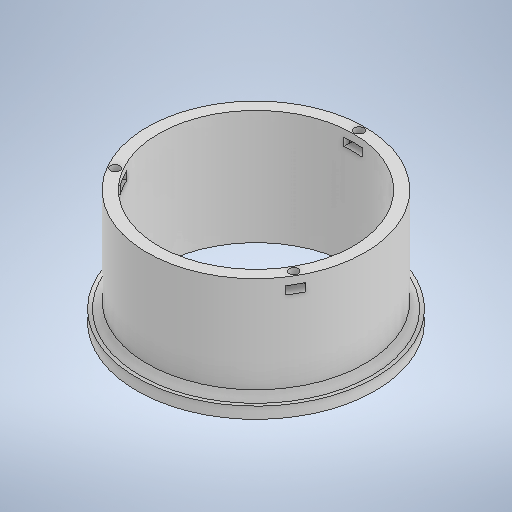
# Autodesk Inventor part: Center Cylinder
Saved by Autodesk Inventor 2025 (Build 290162000, 162)
## iProperties
Created: 2025-07-09
Part Number: Center Cylinder
Material: Generic
Document SubType Name: Modeling
Designer: mumin
Density: 1 g/cm^3
Appearance: Default
Author: mumin
Autodesk Inventor part; units mm, degrees
ref_plane "YZ Plane" through (0, 0, 0) normal (1, 0, 0) x (0, 1, 0)
ref_plane "XZ Plane" through (0, 0, 0) normal (0, 1, 0) x (-1, 0, 0)
ref_plane "XY Plane" through (0, 0, 0) normal (0, 0, 1) x (1, 0, 0)
sketch "Sketch1" plane through (0, 0, 0) normal (0, 0, 1) x (1, 0, 0)
  line L0 (42.5, 0) -> (42.5, 50)
  line L1 (0, -10) -> (0, 60) projected
  line L2 (42.5, 0) -> (52, 0)
  line L3 (52, 0) -> (52, 5)
  line L4 (52, 5) -> (50.5, 5)
  line L5 (47.5, 8) -> (47.5, 50)
  line L6 (-10.4, 0) -> (62.4, 0) projected
  line L7 (50.5, 5) -> (47.5, 8)
  line L8 (42.5, 50) -> (47.5, 50)
  point P0 (0, 0)
  point P1 (47.5, 5)
  point P2 (45, 50)
  dimension "d1" = 5
  dimension "d6" = 3
  dimension "d7" = 3
  dimension "d8" = 50
  dimension "d30" = 9.5
  dimension "d31" = 45
  dimension "d32" = 5
  constraints: 14 end point, 3 perpendicular, 2 horizontal, 2 point on line, 1 midpoint, 1 vertical
  measures "d1" distance of L2.end L3.end
  measures "d6" distance of L4.end point (47.5, 5)
  measures "d7" distance of L5.start point (47.5, 5)
  measures "d8" distance from line of L6 point (45, 50)
  measures "d30" distance of L0.start L2.end
  measures "d31" distance from line of L1 point (45, 50)
  measures "d32" distance of L0.end L5.end
revolve "Revolution1" add sketch "Sketch1" angle 360 about axis through (0, -10, 0) along (0, 1, 0)
ref_plane "Work Plane1" through (0, 45, 0) normal (0, 1, 0) x (1, 0, 0)
sketch "Sketch2" plane through (0, 45, 0) normal (0, 1, 0) x (1, 0, 0)
  arc A0 (-3.996, 44.8222) -> (3.996, 44.8222) centre (0, 0) ccw
  arc A1 (3.996, 44.8222) -> (-3.996, 44.8222) centre (0, 45) ccw
  circle A2 centre (0, 0) radius 42.5 projected
  line L0 (4, 45) -> (4, 41.0512)
  line L1 (4, 41.0512) -> (-4, 41.0512)
  line L2 (-4, 41.0512) -> (-4, 45)
  point P0 (0, 44.7796)
  point P1 (-4, 44.8219)
  point P2 (-4, 42.3113)
  point P3 (4, 42.3113)
  point P4 (4, 44.8219)
  dimension "d11" = 90
  dimension "d12" = 8
  constraints: 6 end point, 6 point on circle, 2 centre point, 1 coincident, 1 parallel
  measures "d11" diameter of A0
  measures "d12" diameter of A1
extrude "Nut Seat" cut sketch "Sketch2" along normal mid plane 3.5 contours A1 A0 L0 A2 L2 | A0 L2 A1 | A0 A1 L0 | L2 L1 L0 A2 | A2 L0 L1 L2
sketch "Sketch3" plane through (0, 50, 0) normal (0, 1, 0) x (1, 0, 0)
  line L0 (0, 72.8) -> (0, -72.8) projected
  point P0 (0, 0)
  point P1 (0, 45)
  dimension "d26" = 45
  constraints: 1 point on line
  measures "d26" distance of point (0, 45) point (0, 0)
hole "Hole1" at (0, 50, -45) direction (0, -1, 0) diameter 4 depth 6.75
pattern_circular "Circular Pattern1" count 3 over 360 about axis through (0, -10, 0) along (0, 1, 0) of "Hole1"
pattern_circular "Circular Pattern2" count 3 over 360 about axis through (0, 25, 0) along (0, 1, 0) of "Nut Seat"
equation "\"d7\" = d6"
body "Solid1"
